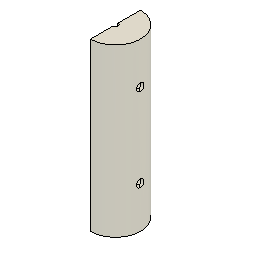
Clicker (Autodesk Fusion 360 archive; units mm, degrees)
design "clicker_a"
Autodesk Fusion 360 part; units mm, degrees
note: some values were not read from the file. Set by a fixed rule: which face or edge a step refers to.
sketch "Sketch1" plane through (0, 0, 0) normal (0, 1, 0) x (1, 0, 0)
  circle A0 centre (0, 0) radius 12
  line L0 (0, -12) -> (0, 12)
  dimension "d1" = 24
  constraint coincident A0.centre origin
  constraint coincident A0 L0.start
  constraint coincident A0 L0.end
  constraint vertical L0
  constraint coincident A0.centre L0
  measures "d1" diameter of A0
extrude "Extrude1" add sketch "Sketch1" along normal blind 80 contours A0 L0 picked at (4.4072, 1.1676)
sketch "Sketch2" plane through (0, 0, 0) normal (0, -1, 0) x (1, 0, 0)
  line L0 (7, -7) -> (-7, -7)
  line L1 (-7, -7) -> (-7, 7)
  line L2 (-7, 7) -> (7, 7)
  line L3 (7, 7) -> (7, -7)
  line L4 (7, -7) -> (-7, 7) construction
  line L5 (-7, -7) -> (7, 7) construction
  line L6 (0, 12) -> (0, -12)
  arc A0 (0, -12) -> (0, 12) centre (0, 0) ccw
  line L7 (0, 12) -> (0, -12)
  dimension "d4" = 14
  dimension "d5" = 14
  constraint horizontal L0
  constraint perpendicular L0 L1
  constraint parallel L0 L2
  constraint parallel L1 L3
  constraint coincident L4 A0.centre
  constraint coincident L5 A0.centre
  constraint coincident A0.centre origin
  constraint coincident L6.start A0
  constraint coincident L6.end A0
  constraint perpendicular L0 L6
  constraint coincident A0.centre L6
  measures "d4" distance of L1.end L2.end
  measures "d5" distance of L0.end L1.end
shell "Shell1" thickness 3 removed faces 1 at (0, 53.3333, 4)
extrude "Extrude2" cut sketch "Sketch2" against normal up to surface (3 mm away) contours L0 L2 L3 L6 L7 | L0 L1 L2 L6 L7
sketch "Sketch6" plane through (0, 0, 0) normal (0, -1, 0) x (1, 0, 0)
  line L0 (0, 7) -> (7, 7)
  line L1 (7, 7) -> (7, -7)
  line L2 (7, -7) -> (0, -7)
  line L3 (0, -7) -> (0, -12)
  arc A0 (0, -12) -> (0, 12) centre (0, 0) ccw
  line L4 (0, 12) -> (0, 7)
  arc A1 (5.6569, 7) -> (0, 9) centre (0, 0) ccw
  arc A2 (0, -9) -> (0, 9) centre (0, 0) ccw
  arc A3 (0, -9) -> (5.6569, -7) centre (0, 0) ccw
  arc A4 (5.6569, -7) -> (7, -5.6569) centre (0, 0) ccw
  arc A5 (7, -5.6569) -> (7, 5.6569) centre (0, 0) ccw
  arc A6 (7, 5.6569) -> (5.6569, 7) centre (0, 0) ccw
  line L5 (8.8824, -1.45) -> (8.8824, 1.45)
  dimension "d25" = 2.9
  constraint coincident A2 L5.start
  constraint coincident A5 L5.start
  constraint coincident A2 L5.end
  constraint vertical L5
  measures "d25" distance of L5.start L5.end
extrude "Extrude6" add sketch "Sketch6" against normal blind 77 contours A2 A5 L5
sketch "Sketch3" plane through (0, 80, 0) normal (0, 1, 0) x (-1, 0, 0)
  arc A0 (0, 12) -> (0, -12) centre (0, 0) ccw
  line L0 (0, -12) -> (0, 12)
  circle A1 centre (0, 0) radius 1.2
  dimension "d9" = 2.4
  constraint coincident A0.centre A1.centre
  measures "d9" diameter of A1
extrude "Extrude3" cut sketch "Sketch3" against normal up to surface (3 mm away) contours L0 A1 picked at (-0.3723, -0.1461)
ref_plane "WorkPlane1" through (12, 40, 0) normal (1, 0, 0) x (0, 0, -1)
sketch "Sketch4" plane through (12, 0, 0) normal (1, 0, 0) x (0, 0, -1)
  circle A0 centre (0, 60) radius 1
  line L0 (12, 80) -> (-12, 80)
  line L1 (0, 80) -> (0, 0) construction
  circle A1 centre (0, 20) radius 1
  line L2 (12, 0) -> (-12, 0) construction
  dimension "d13" = 2
  dimension "d14" = 20
  dimension "d15" = 2
  dimension "d16" = 20
  constraint midpoint L0 L1.start
  constraint coincident L1.end origin
  constraint coincident A0.centre L1
  constraint coincident L1 A1.centre
  measures "d13" diameter of A0
  measures "d14" distance of A0.centre L0
  measures "d15" diameter of A1
  measures "d16" distance of A1.centre L2
extrude "Extrude4" cut sketch "Sketch4" against normal blind 45
chamfer "Chamfer1" distance 0.8 angle 45 4 edges at (11.9583, 20, -1) (11.9583, 20, 1) (11.9583, 60, -1) (11.9583, 60, 1)

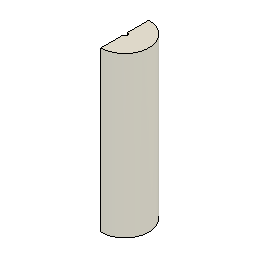
design "clicker_b"
Autodesk Fusion 360 part; units mm, degrees
sketch "Sketch1" plane through (0, 0, 0) normal (0, 1, 0) x (1, 0, 0)
  circle A0 centre (0, 0) radius 12
  line L0 (0, -12) -> (0, 12)
  circle A1 centre (0, 0) radius 9
  line L1 (-8.8824, 1.45) -> (-8.8824, -1.45)
  line L2 (-9, 3) -> (9, 3)
  line L3 (9, 3) -> (9, -3)
  line L4 (9, -3) -> (-9, -3)
  line L5 (-9, -3) -> (-9, 3)
  line L6 (-9, 3) -> (9, -3) construction
  line L7 (9, 3) -> (-9, -3) construction
  dimension "d1" = 24
  dimension "d33" = -3
  dimension "d34" = 2.9
  dimension "d35" = 6
  constraint coincident A0.centre A1.centre
  constraint coincident A0 L0.start
  constraint coincident A0 L0.end
  constraint vertical L0
  constraint coincident A0.centre L0
  constraint coincident A1 L1.start
  constraint coincident A1 L1.end
  constraint vertical L1
  constraint horizontal L2
  constraint perpendicular L2 L3
  constraint parallel L2 L4
  constraint parallel L3 L5
  constraint coincident L6 A0.centre
  constraint coincident L7 A0.centre
  constraint tangent A1 L5
  measures "d1" diameter of A0
  measures "d34" distance of L1.start L1.end
  measures "d35" distance of L2.end L3.end
extrude "Extrude1" add sketch "Sketch1" along normal blind 80 contours A0 L0 A1 L2 L3 L4 | L0 A1 L2 | L0 A1 L4 | L0 A1 L2 L4 | A1 L2 L3 | A1 L3 L4 picked at (0.409, 6.972) picked at (0.409, -6.972)
sketch "Sketch2" plane through (0, 0, 0) normal (0, -1, 0) x (1, 0, 0)
  line L0 (7, -7) -> (-7, -7)
  line L1 (-7, -7) -> (-7, 7)
  line L2 (-7, 7) -> (7, 7)
  line L3 (7, 7) -> (7, -7)
  line L4 (7, -7) -> (-7, 7) construction
  line L5 (-7, -7) -> (7, 7) construction
  line L6 (0, 12) -> (0, -12)
  arc A0 (0, -12) -> (0, 12) centre (0, 0) ccw
  line L7 (0, 12) -> (0, -12)
  dimension "d4" = 14
  dimension "d5" = 14
  constraint horizontal L0
  constraint perpendicular L0 L1
  constraint parallel L0 L2
  constraint parallel L1 L3
  constraint coincident L4 A0.centre
  constraint coincident L5 A0.centre
  constraint coincident A0.centre origin
  constraint coincident L6.start A0
  constraint coincident L6.end A0
  constraint perpendicular L0 L6
  constraint coincident A0.centre L6
  measures "d4" distance of L1.end L2.end
  measures "d5" distance of L0.end L1.end
shell "Shell1" thickness 3 removed faces 5 at (0, 26.6667, -10) at (0, 26.6667, -5) at (0, 26.6667, 1) at (0, 26.6667, 7) at (0, 26.6667, 11)
extrude "Extrude2" cut sketch "Sketch2" against normal up to surface (3 mm away) contours L0 L2 L3 L6 L7 | L0 L1 L2 L6 L7
sketch "Sketch3" plane through (0, 80, 0) normal (0, 1, 0) x (-1, 0, 0)
  arc A0 (0, 12) -> (0, -12) centre (0, 0) ccw
  line L0 (0, -12) -> (0, 12)
  circle A1 centre (0, 0) radius 1.2
  dimension "d9" = 2.4
  constraint coincident A0.centre A1.centre
  measures "d9" diameter of A1
extrude "Extrude3" cut sketch "Sketch3" against normal up to surface (3 mm away) contours L0 A1 picked at (-0.3723, -0.1461)
ref_plane "WorkPlane2" through (9, 40, 0) normal (1, 0, 0) x (0, 0, -1)
sketch "Sketch5" plane through (9, 0, 0) normal (1, 0, 0) x (0, 0, -1)
  line L0 (5.6569, 3) -> (7, 3)
  line L1 (7, 3) -> (7, 0)
  line L2 (7, 0) -> (-7, 0)
  line L3 (-7, 0) -> (-7, 3)
  line L4 (-7, 3) -> (-5.6569, 3)
  line L5 (-5.6569, 3) -> (5.6569, 3)
  line L6 (1.2, 77) -> (-1.2, 77)
  line L7 (-1.2, 77) -> (-1.2, 80)
  line L8 (-1.2, 80) -> (1.2, 80)
  line L9 (1.2, 80) -> (1.2, 77)
  line L10 (0, 80) -> (0, 0) construction
  circle A0 centre (0, 60) radius 3
  circle A1 centre (0, 20) radius 3
  dimension "d21" = 6
  dimension "d22" = 6
  dimension "d23" = 20
  dimension "d24" = 20
  constraint midpoint L8 L10.start
  constraint coincident L10.end origin
  constraint coincident L10 A0.centre
  constraint coincident L10 A1.centre
  measures "d21" diameter of A0
  measures "d22" diameter of A1
  measures "d23" distance of L8 A0.centre
  measures "d24" distance of L2 A1.centre
extrude "Extrude5" add sketch "Sketch5" against normal blind 18 contours A0 | A1
sketch "Sketch6" plane through (-9, 0, 0) normal (-1, 0, 0) x (0, 0, 1)
  circle A0 centre (0, 60) radius 3
  circle A1 centre (0, 60) radius 1.45
  circle A2 centre (0, 20) radius 1.45
  circle A3 centre (0, 20) radius 3
  dimension "d27" = 2.9
  dimension "d28" = 2.9
  constraint concentric A0 A1
  constraint concentric A2 A3
  measures "d27" diameter of A1
  measures "d28" diameter of A2
extrude "Extrude6" cut sketch "Sketch6" against normal blind 5 contours A1 | A2
fillet "Fillet1" radius 2 4 edges at (8.4853, 20, 3) (8.4853, 20, -3) (8.4853, 60, -3) (8.4853, 60, 3)
extrude "Extrude7" cut sketch "Sketch1" along normal blind 90 contours A1 L2 L5 | A1 L4 L5 | A1 L1
ref_plane "WorkPlane1" through (12, 40, 0) normal (1, 0, 0) x (0, 0, -1)
sketch "Sketch4" plane through (12, 0, 0) normal (1, 0, 0) x (0, 0, -1)
  circle A0 centre (0, 72) radius 1
  line L0 (12, 80) -> (-12, 80)
  line L1 (0, 80) -> (0, 0) construction
  circle A1 centre (0, 8) radius 1
  line L2 (12, 0) -> (-12, 0) construction
  dimension "d13" = 2
  dimension "d14" = 8
  dimension "d15" = 2
  dimension "d16" = 8
  constraint midpoint L0 L1.start
  constraint coincident L1.end origin
  constraint coincident A0.centre L1
  constraint coincident L1 A1.centre
  measures "d13" diameter of A0
  measures "d14" distance of A0.centre L0
  measures "d15" diameter of A1
  measures "d16" distance of A1.centre L2
extrude "Extrude4" [rolled back] side1offset 0 taper angle 0
chamfer "Chamfer1" [rolled back] distance 0.8
